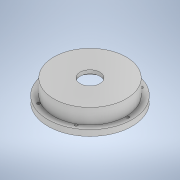
# Autodesk Inventor part: Stage_1_Lid
Saved by Autodesk Inventor 2022.3 (Build 263350000, 350)
## iProperties
Created: 2022-05-21
Part Number: Stage_1_Lid
Material: Generic
Document SubType Name: Modeling
Designer: Mlees
Density: 1 g/cm^3
Appearance: Aluminum - Polished
Author: Mlees
Autodesk Inventor part; units mm, degrees
ref_plane "YZ Plane" through (0, 0, 0) normal (1, 0, 0) x (0, 1, 0)
ref_plane "XZ Plane" through (0, 0, 0) normal (0, 1, 0) x (-1, 0, 0)
ref_plane "XY Plane" through (0, 0, 0) normal (0, 0, 1) x (1, 0, 0)
sketch "Sketch1" plane through (0, 0, 0) normal (0, 1, 0) x (-1, 0, 0)
  circle A0 centre (0, 0) radius 36
  circle A1 centre (0, 0) radius 29
  line L0 (0, 0) -> (32.313, 0)
  circle A2 centre (32.313, 0) radius 1.25
  circle A3 centre (16.1565, 27.9839) radius 1.25
  circle A4 centre (-16.1565, 27.9839) radius 1.25
  circle A5 centre (-32.313, 0) radius 1.25
  circle A6 centre (-16.1565, -27.9839) radius 1.25
  circle A7 centre (16.1565, -27.9839) radius 1.25
  dimension "d0" = 72
  dimension "d1" = 58
  dimension "d2" = 32.313
  dimension "d3" = 2.5
  dimension "d6" = 360
  constraints: 8 centre point, 3 coincident, 2 end point, 1 horizontal, 13 other
  measures "d0" diameter of A0
  measures "d1" diameter of A1
  measures "d2" distance of L0.start L0.end
  measures "d3" diameter of A2
extrude "Extrusion1" add sketch "Sketch1" along normal blind 15
sketch "Sketch2" plane through (0, 15, 0) normal (0, 1, 0) x (1, 0, 0)
  circle A0 centre (0, 0) radius 29
  circle A1 centre (0, 0) radius 31.063
  circle A2 centre (-16.1565, 27.9839) radius 1.25 projected
  circle A3 centre (0, 0) radius 36
  point P0 (-15.5315, 26.9013)
  constraints: 3 centre point, 3 coincident, 1 tangent
extrude "Extrusion2" cut sketch "Sketch2" against normal blind 10 contours A3
sketch "Sketch3" plane through (0, 15, 0) normal (0, 1, 0) x (1, 0, 0)
  circle A0 centre (0, 0) radius 31.063
  circle A1 centre (0, 0) radius 8.5
  dimension "d12" = 17
  constraints: 2 centre point, 2 coincident
  measures "d12" diameter of A1
extrude "Extrusion3" add sketch "Sketch3" along normal blind 3
body "Solid1"
